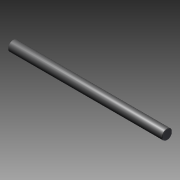
# Autodesk Inventor part: SSFHR12-185_s
Saved by Autodesk Inventor 2011 SP1 (Build 150282100, 282)
## iProperties
Created: 2016-04-11
Part Number: SSFHR12-185_s
Catalog Web Link: www.cadenas.de
Description: SFMR, PSFMR, SSFMR, SFHR, PSFHR, SSFHR, SFR, PSFR, SSFR, HFR, PHFR_shaft-Rotary Shafts - Straight -
Vendor: MISUMI
Document SubType Name: Modeling
Designer: psAdmin
Manufacturer: MISUMI
Mass: 20.9138 g
Surface Area: 71.778 cm^2
Volume: 20.9138 cm^3
Density: 1 g/cm^3
Category: PARTsolutions
Company: MISUMI
Title: SSFHR12-185
Author: Cadenas PARTsolutions
Comments: Rotary Shafts - Straight -
PSOL_IDENT_0: {$CADENAS_DATA\23d-libs\misumi\metric\11_rotary_shafts\11_components\psfr\psfr.prj},371 {VTYP=3D},{N
PSOL_IDENT_1: B=SSFHR12-185_s},{LINA=SSFHR12-185},{NN=SFMR, PSFMR, SSFMR, SFHR, PSFHR, SSFHR, SFR, PSFR, SSFR, HFR
PSOL_IDENT_2: , PHFR_shaft},{DATE=27.10.2015 07:30:26},{GEOMDATE=20.10.2015 04:49:10},{VERSION=},{LINEID=40},{LINE
PSOL_IDENT_3: SUBID=-1},{WBVAR=TS,MAT,ST,ALT1,L,ALT2,KC,A,WKC,C,K,E,KZ,Z,ALT3,FC,GALT3,WFC,J,WALT3,V,ALT4,SFC,SG,A
PSOL_IDENT_4: G,ALT10,KWC,ALT11,WC,ALT6,TA,TB,ALT5,UC,ALT7,SC,ALT32,CD}  {NB=SSFHR12-185_s},{LINA=SSFHR12-185},{KT=
PSOL_IDENT_5: DUMMY},{PN=SSFHR12-185},{TYPE=SSFHR},{TS=H},{TSALG='M','h9 (Cold-drawn)','H','h7 (Ground)','','g6 (G
PSOL_IDENT_6: round)'},{MAT=SUS304},{MATALG= 'S45C','S45C Equivalent', 'SUS304','SUS304' },{ST=-},{STALG= '-','-'
PSOL_IDENT_7: },{D=12.0},{ALT1=},{L=185.0},{LALG=[15:700/0.1]},{LMIN=15},{LMAX=700},{ALT2=},{ALT2ALG= '', 'w/o Key
PSOL_IDENT_8: Grooves','KC','with KC (Key Groove)','WKC','with WKC (Two Key Grooves)','KCWKC','with KC + WKC (Thr
PSOL_IDENT_9: ee Key Grooves)','KZ','with KC + WKC + KZ (Four Key Grooves)' },{ALT2PN=},{KC=0.0},{KCALG=[0]},{KCMI
PSOL_IDENT_10: N=0},{KCMAX=181},{KCMIN1=0},{KCMIN2=4},{KCMIN3=8},{KCMIN4=12},{KCMAX1=169},{KCMAX2=173},{KCMAX3=177}
PSOL_IDENT_11: ,{KCMAX4=181},{A=0.0},{AALG=[0]},{AMIN=4},{AMAX=100},{AMAX1=100},{AMAX2=100},{AMAX3=100},{AMAX4=100}
PSOL_IDENT_12: ,{WKC=0.0},{WKCALG=[0]},{WKCMIN=0},{WKCMIN1=0},{WKCMIN2=0},{WKCMIN3=0},{WKCMIN4=0},{WKCMAX=177},{WKC
PSOL_IDENT_13: MAX1=0},{WKCMAX2=0},{WKCMAX4=177},{WKCMINKZ1=0},{WKCMAXKZ1=-4},{WKCMINKZ2=0},{WKCMAXKZ2=177},{WKCMIN
PSOL_IDENT_14: KZ3=4},{WKCMAXKZ3=-8},{WKCMINKZ4=4},{WKCMAXKZ4=-4},{WKCMAXKZ5=-8},{WKCMINKZ6=-8},{WKCMAXKZ6=185},{WK
PSOL_IDENT_15: CMINKZ7=185},{WKCMAXKZ7=173},{C=0.0},{CALG=[0]},{CMIN=4},{CMAX=0},{CMAX1=100},{CMAX2=0},{CMAX3=-4},{
PSOL_IDENT_16: CMAX4=-4},{CMAX5=-8},{K=0.0},{KALG=[0]},{KMIN=0},{KMIN1=0},{KMIN2=185},{KMIN3=4},{KMIN4=189},{KMAX=1
PSOL_IDENT_17: 81},{KMAX1=181},{KMAX2=181},{KMAX3=181},{KMAX4=177},{E=0.0},{EALG=[0]},{EMIN=4},{EMAX=100},{EMAX1=10
PSOL_IDENT_18: 0},{EMAX2=100},{EMAX3=100},{EMAX4=100},{KZ=0.0},{KZALG=[0]},{KZMIN1=0},{KZMIN2=0},{KZMIN3=0},{KZMIN4=
PSOL_IDENT_19: 185},{KZMAX1=-4},{KZMAX2=-4},{KZMAX3=181},{KZMAX4=181},{KZMINL1=0},{KZMINL2=0},{KZMINL3=0},{KZMINL4=
PSOL_IDENT_20: 185},{KZMINC1=0},{KZMINC2=0},{KZMINC3=0},{KZMINC4=185},{KZMINR1=0},{KZMINR2=0},{KZMINR3=185},{KZMINR
PSOL_IDENT_21: 4=0},{KZMAXL1=-4},{KZMAXL2=-4},{KZMAXL3=181},{KZMAXL4=181},{KZMAXC1=-4},{KZMAXC2=-4},{KZMAXC3=181},{
PSOL_IDENT_22: KZMAXC4=181},{KZMAXR1=-4},{KZMAXR2=181},{KZMAXR3=-4},{KZMAXR4=181},{Z=0.0},{ZALG=[0]},{ZMIN=4},{ZMAX=
PSOL_IDENT_23: 0},{ZMAX1=0},{ZMAX2=100},{ZMAX3=100},{BB=4},{TT=2.5},{CIFKC=0},{CIFWKC=0},{CIFK=0},{CIFKZ=0},{CIF2BB=
PSOL_IDENT_24: 0},{CIF1BBA=13},{CIF1BBB=0},{CIF1BBC=45},{CIF1BBKC=1},{CIF1BBWKC=1},{CIF1BBK=2},{CIF2BBA=0},{CIF2BBB=
PSOL_IDENT_25: 60},{CIF2BBC=92},{CIF2BBD=0},{CIF2BBE=156},{CIF2BBF=188},{CIF2BBG=0},{CIF2BBH=0},{CIF2BBI=0},{CIF2BB
PSOL_IDENT_26: J=316},{CIF2BBK=348},{CIF2BBL=0},{CIFBBKC=1},{CIFBBWKC=1},{CIFBBK=2},{CIFBBKZ=1},{CIFWKC1=0},{ALT3=}
PSOL_IDENT_27: ,{ALT3ALG= '', 'w/o Set Screw Flat','FC','with FC (Adds a Set Screw Flat)','WFC','with WFC (Adds Two
PSOL_IDENT_28: Set Screw Flats)','FCWFC','with FC + WFC (Adds Three Set Screw Flats)' },{ALT3PN=},{FC=0},{FCALG=[0
PSOL_IDENT_29: ]},{FCMIN=0},{FCMAX=184},{GALT3=0},{GALT3ALG=[0]},{GALT3MIN=1},{GALT3MAX=70},{GALT3MAX2=70},{GALT3MA
PSOL_IDENT_30: X3=70},{WFC=0},{WFCALG=[0]},{WFCMIN=0},{WFCMIN2=2},{WFCMAX=181},{WFCMAX2=-3},{WFCMAX3=-4},{J=0},{JAL
PSOL_IDENT_31: G=[0]},{JMIN=1},{JMAX=70},{JMAX2=-2},{JMAX3=-5},{WALT3=0},{WALT3ALG=[0]},{WALT3MIN=0},{WALT3MIN2=187
PSOL_IDENT_32: },{WALT3MAX=182},{WALT3MAX2=182},{WALT3MAX3=182},{V=0},{VALG=[0]},{VMIN=1},{VMAX=70},{VMAX2=70},{VMA
PSOL_IDENT_33: X3=50},{CIFFC=0},{ALT4=},{ALT4ALG= '', 'w/o SFC (2 Set Screw Flats (Angle Specified))', 'SFC'  , 'wi
PSOL_IDENT_34: th SFC (2 Set Screw Flats (Angle Specified))'},{ALT4PN=},{SFC=0},{SFCALG=[0]},{SFCMIN=0},{SFCMAX=184
PSOL_IDENT_35: },{SG=0},{SGALG=[0]},{SGMIN=1},{SGMAX=70},{AG=0},{AGALG=[0]},{H=0.0},{CIFSFC=0},{ALT10=},{ALT10ALG= ''
PSOL_IDENT_36: , 'w/o KWC (2 Set Screw Flats at both ends)', 'KWC', 'with KWC (2 Set Screw Flats at both ends)' },{
PSOL_IDENT_37: ALT10PN=},{KWC=0},{KWCALG=[0]},{KWCMIN=1},{KWCMAX=91.5},{WALT10=9},{ALT11=},{ALT11ALG= '','Not appli
PSOL_IDENT_38: cable' },{ALT11PN=},{WC=0.0},{WCALG=[0]},{ALT6=},{ALT6ALG= '','w/o Retaining Ring Groove','TA','with
PSOL_IDENT_39: TA (Retaining Ring Groove)','TB','with TB (Retaining Ring Groove)','TATB','with TA + TB (Two Retain
PSOL_IDENT_40: ing Ring Grooves)' },{ALT6PN=},{TA=0.0},{TAALG=[0]},{TAMIN=2},{TAMAX=0},{TB=0.0},{TBALG=[0]},{TBMIN=
PSOL_IDENT_41: 2},{TBMAX=0},{DDALT6=0.0},{MM=0.00},{ALT5=},{ALT5ALG= '', 'w/o UC (Slit Cam Groove)', 'UC', 'with UC
PSOL_IDENT_42: (Slit Cam Groove)'},{ALT5PN=},{UC=0},{UCALG=[0]},{UCMIN=1},{UCMAX=179},{DDALT5=0},{LL1=0},{ALT7=},{
PSOL_IDENT_43: ALT7ALG= '', 'w/o SC (Wrench Flats)', 'SC', 'with SC (Wrench Flats)'},{ALT7PN=},{SC=0},{SCALG=[0]},{
PSOL_IDENT_44: SCMIN=0},{SCMAX=175},{WALT7=0},{LL2=0},{LL2ALG=10},{CIFSC=0},{ALT32=},{ALT32ALG=  '','w/o CD (Change
PSOL_IDENT_45: s Part D Chamfering)','-CD', 'with CD (Changes Part D Chamfering)' },{ALT32PN=},{CD=},{CDALG= '','N/
PSOL_IDENT_46: A' },{CD3D=0.5},{CIF32=0},{CIF320=0},{CIFTA=0},{CIFTB=0},{ERRORPN=},{ERRORALT23=OK},{ERRORALT24=OK},
PSOL_IDENT_47: {ERRORALT25=OK},{ERRORALT26=OK},{ERRORALT27=OK},{ERRORALT210=OK},{ERRORALT34=OK},{ERRORALT35=OK},{ER
PSOL_IDENT_48: RORALT36=OK},{ERRORALT37=OK},{ERRORALT310=OK},{ERRORALT45=OK},{ERRORALT46=OK},{ERRORALT47=OK},{ERROR
PSOL_IDENT_49: ALT410=OK},{ERRORALT56=OK},{ERRORALT57=OK},{ERRORALT510=OK},{ERRORALT610=OK},{ERRORALT75=OK},{ERRORA
PSOL_IDENT_50: LT76=OK},{ERRORALT710=OK}
NN: SFMR, PSFMR, SSFMR, SFHR, PSFHR, SSFHR, SFR, PSFR, SSFR, HFR, PHFR_shaft
NT: Rotary Shafts - Straight -
NB: SSFHR12-185_s
NBSYN: $PN._s
LINA: SSFHR12-185
PN: SSFHR12-185
TS: h7 (Ground)
MAT: SUS304
ST: -
D: 12.0
ALT1: w/o LKC (Changes L Tolerance)
L: 185.0
ALT2: w/o Key Grooves
KC: 0.0
A: 0.0
WKC: 0.0
C: 0.0
K: 0.0
E: 0.0
KZ: 0.0
Z: 0.0
ALT3: w/o Set Screw Flat
FC: 0
GALT3: 0
WFC: 0
J: 0
WALT3: 0
V: 0
ALT4: w/o SFC (2 Set Screw Flats (Angle Specified))
SFC: 0
SG: 0
AG: 0
H: 0.0
ALT10: w/o KWC (2 Set Screw Flats at both ends)
KWC: 0
ALT11: Not applicable
WC: 0.0
ALT6: w/o Retaining Ring Groove
TA: 0.0
TB: 0.0
DDALT6: 0.0
MM: 0.00
ALT5: w/o UC (Slit Cam Groove)
UC: 0
DDALT5: 0
LL1: 0
ALT7: w/o SC (Wrench Flats)
SC: 0
WALT7: 0
LL2: 0
ALT32: w/o CD (Changes Part D Chamfering)
CD: N/A
SUPPLIER: MISUMI
ARTICLENO: SSFHR12-185_s
BOMINFO: SSFHR12-185
CREATOR: CADENAS GmbH
Autodesk Inventor part; units mm, degrees
sketch "Sketch_1" plane through (0, 0, 0) normal (0, 0, 1) x (1, 0, 0)
  line L0 (185, 0) -> (0, 0)
  line L1 (0, 0) -> (0, 5.5)
  line L2 (0, 5.5) -> (0.5, 6)
  line L3 (0.5, 6) -> (184.5, 6)
  line L4 (184.5, 6) -> (185, 5.5)
  line L5 (185, 5.5) -> (185, 0)
  line L6 (185, 0) -> (0, 0)
  constraints: 14 end point
revolve "Revolution1" add sketch "Sketch_1" angle 360 about axis through (185, 0, 0) along (1, 0, 0)
ref_plane "COMBINATION_MODULE_XY" through (0, 0, 0) normal (1, 0, 0) x (0, 0, -1)
ref_plane "COMBINATION_MODULE_YZ" through (0, 0, 0) normal (0, 0, -1) x (0, 1, 0)
ref_plane "COMBINATION_MODULE_ZX" through (0, 0, 0) normal (0, 1, 0) x (1, 0, 0)
body "Solid1"
